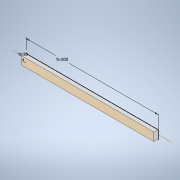
# Autodesk Inventor part: track_walls
Saved by Autodesk Inventor 2021 (Build 250183000, 183)
## iProperties
Created: 2021-02-13
Part Number: track_walls
Material: Generic
Document SubType Name: Modeling
Designer: phamv
Density: 1 g/cm^3
Appearance: Default
Author: phamv
Autodesk Inventor part; units mm, degrees
ref_plane "YZ Plane" through (0, 0, 0) normal (1, 0, 0) x (0, 1, 0)
ref_plane "XZ Plane" through (0, 0, 0) normal (0, 1, 0) x (-1, 0, 0)
ref_plane "XY Plane" through (0, 0, 0) normal (0, 0, 1) x (1, 0, 0)
sketch "Sketch1" plane through (0, 0, 0) normal (0, 0, 1) x (1, 0, 0)
  line L0 (-400, 25) -> (400, 25)
  line L1 (400, 25) -> (400, -25)
  line L2 (400, -25) -> (-400, -25)
  line L3 (-400, -25) -> (-400, 25)
  line L4 (0, -25) -> (0, 25) construction
  point P0 (0, 0)
  point P1 (0, 0)
  dimension "d0" = 800
  dimension "d1" = 50
  constraints: 10 end point, 3 midpoint, 2 parallel, 1 coincident, 1 horizontal, 1 perpendicular
  measures "d0" distance between parallel lines of L1 L3
  measures "d1" distance between parallel lines of L2 L0
extrude "Extrusion1" add sketch "Sketch1" along normal blind 25
equation "\"d0\" = wall_length"
equation "\"d1\" = wall_width"
equation "\"d2\" = wall_thickness"
equation "\"edge_gap_distance\" = 14.5"
equation "\"wall_length\" = 800"
equation "\"wall_width\" = -0.5 * track_width + 0.5 * layer_width"
equation "\"wall_thickness\" = 25"
equation "\"p_______________________________________\" = 1"
equation "\"track_width\" = 300"
equation "\"layer_width\" = 400"
body "Solid1"
